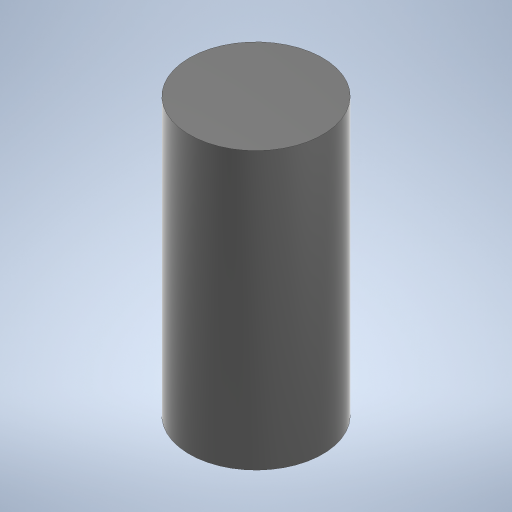
# Autodesk Inventor part: movil_llanta
Saved by Autodesk Inventor 2024 (Build 280153000, 153)
## iProperties
Created: 2023-05-06
Part Number: movil_llanta
Material: Generic
Document SubType Name: Modeling
Designer: Diego
Density: 1 g/cm^3
Appearance: Default
Author: Diego
Autodesk Inventor part; units mm, degrees
ref_plane "YZ Plane" through (0, 0, 0) normal (1, 0, 0) x (0, 1, 0)
ref_plane "XZ Plane" through (0, 0, 0) normal (0, 1, 0) x (-1, 0, 0)
ref_plane "XY Plane" through (0, 0, 0) normal (0, 0, 1) x (1, 0, 0)
sketch "Sketch1" plane through (0, 0, 0) normal (0, 1, 0) x (-1, 0, 0)
  circle A0 centre (0, 0) radius 6.5
  dimension "d0" = 13
  constraints: 1 centre point, 1 coincident
  measures "d0" diameter of A0
extrude "Extrusion1" add sketch "Sketch1" along normal blind 27
ref_plane "Work Plane1" through (-15.9078, 0, 6.5) normal (1, 0, 0) x (0, 0, -1)
sketch "Sketch4" plane through (-15.9078, 0, 6.5) normal (1, 0, 0) x (0, 0, -1)
  line L0 (6.5, 0) -> (6.5, 27) construction
  line L1 (13, 27) -> (0, 27) construction
  circle A0 centre (6.5, 13.5) radius 3.75
  dimension "d9" = 7.5
  constraints: 2 end point, 2 midpoint, 1 centre point
  measures "d9" diameter of A0
extrude "Extrusion3" cut sketch "Sketch4" along normal blind 18
body "Solid1"
